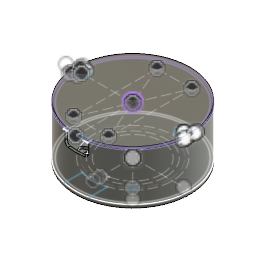
Pixelmapping_gehaeuse (Autodesk Fusion 360 design; units mm, degrees)
Autodesk Fusion 360 part; units mm, degrees
sketch "LED-Ring" plane through (0, 0, 0) normal (0, 1, 0) x (1, 0, 0)
  circle A0 centre (0, 0) radius 18
  circle A1 centre (0, 0) radius 20.7 construction
  line L0 (0, 0) -> (0, -20.7) construction
  line L1 (2.8, -17.9) -> (-2.8, -17.9)
  line L2 (-2.8, -17.9) -> (-2.8, -23.5)
  line L3 (-2.8, -23.5) -> (2.8, -23.5)
  line L4 (2.8, -23.5) -> (2.8, -17.9)
  line L5 (2.8, -17.9) -> (-2.8, -23.5) construction
  line L6 (-2.8, -17.9) -> (2.8, -23.5) construction
  circle A2 centre (0, -20.7) radius 1.75
  line L7 (0, 0) -> (22.6032, -22.6032) construction
  line L8 (0, 0) -> (31.9658, 0) construction
  circle A3 centre (0, 0) radius 23.18 construction
  circle A4 centre (16.3907, -16.3907) radius 1.25
  circle A5 centre (0, 0) radius 36
  circle A6 centre (16.3907, -16.3907) radius 2.25
  line L9 (7.9114, -23.7152) -> (7.9114, -35.1199)
  line L10 (-7.9114, -35.1199) -> (-7.9114, -23.7152)
  arc A7 (-7.9114, -23.7152) -> (7.9114, -23.7152) centre (0, 0) ccw
  arc A8 (17.6777, -17.6777) -> (16.6799, -18.6221) centre (0, 0) ccw
  line L11 (-2.8, -23.5) -> (2.8, -23.5)
  line L12 (2.8, -23.5) -> (2.8, -25.3)
  line L13 (2.8, -25.3) -> (-2.8, -25.3)
  line L14 (-2.8, -25.3) -> (-2.8, -23.5)
  circle A9 centre (0, 0) radius 34.5
  point P0 (0, -20.7)
  point P1 (0, -25)
  dimension "d170" = 50
  dimension "d171" = 36
  dimension "d172" = 2.7
  dimension "d173" = 5.6
  dimension "d174" = 5.6
  dimension "d175" = 3.5
  dimension "d176" = 45
  dimension "d178" = 2.5
  dimension "d179" = 72
  dimension "d190" = 4.5
  dimension "d267" = 1.8
  dimension "d308" = 69
  constraint coincident A0.centre A1.centre
  constraint concentric A0 A8
  constraint coincident A1 P0
  constraint vertical L0
  constraint horizontal L1
  constraint perpendicular L1 L2
  constraint parallel L1 L3
  constraint parallel L2 L4
  constraint coincident L5 P0
  constraint coincident L6 P0
  constraint coincident P0 L0.end
  constraint horizontal L8
  constraint coincident L7 A4.centre
  constraint coincident A3 A4.centre
  constraint concentric A5 A8
  constraint concentric A4 A6
  constraint parallel L9 L10
  constraint coincident P1 A8
  constraint coincident L9.start A8
  constraint coincident L10.end A8
  constraint coincident A5 L10.start
  constraint coincident A5 L9.end
  constraint coincident A6 A8.end
  constraint concentric A3 A8
  constraint coincident L7 A8.start
  constraint horizontal L11
  constraint vertical L12
  constraint horizontal L13
  constraint vertical L14
  constraint concentric A5 A9
  measures "d170" diameter of A8
  measures "d171" diameter of A0
  measures "d173" distance of L2.end L3.end
  measures "d174" distance of L1.end L2.end
  measures "d175" diameter of A2
  measures "d176" angle of L7 L8
  measures "d178" diameter of A4
  measures "d179" diameter of A5
  measures "d190" diameter of A6
  measures "d267" distance of L2.end L13.end
  measures "d308" diameter of A9
extrude "LED-Ring Base Plate" add sketch "LED-Ring" against normal blind 2 contours A0 L1 | A0 L1 L2 L4 A6 A7 A8 L12 L14 | A0 L1 | A0 L1 L2 L3 L4 L11 | L3 A7 A8 L11 L12 L14 | L9 L10 A7 A8 L12 L13 L14 A9 | A7 A8 L12 L13 L14 | A6 L9 L10 A8 A9 | A5 L9 L10 A9 | A5 L9 L10 A9 | A6 | A2 | A4 makes body 1
extrude "Lichtloch" cut sketch "LED-Ring" against normal blind 2 contours A2 bodies 1
pattern_circular "Löcher Lattern" count 12 over 360 about axis through (0, 0, 0) along (0, 1, 0) of "Lichtloch"
extrude "SMD Loch" cut sketch "LED-Ring" against normal blind 1.5 contours A0 L1 | A0 L1 L2 L3 L4 L11 | L3 A7 A8 L11 L12 L14 | A7 A8 L12 L13 L14 picked at (-0.2109, -17.9296) bodies 1
fillet "Fillet4" radius 1.6 2 edges at (2.8, -0.75, 25.3) (-2.8, -0.75, 25.3) on bodies 1
pattern_circular "SMD Aussparungen" count 12 over 360 about axis through (0, 0, 0) along (0, 1, 0) of "SMD Loch", "Fillet4"
extrude "Schraubenloch" cut sketch "LED-Ring" against normal blind 5 contours A4 bodies 1
chamfer "Chamfer4" distance 1 angle 45 1 edges at (15.2253, -2, 16.8428) on bodies 1
pattern_circular "C-Pattern3" count 4 over 360 about axis through (0, 0, 0) along (0, 1, 0) of "Schraubenloch", "Chamfer4"
extrude "Extrude21" cut sketch "LED-Ring" against normal blind 1.4 contours L9 L10 A7 A8 L12 L13 L14 A9 | A7 A8 L12 L13 L14 | A5 L9 L10 A9 picked at (2.2129, -34.8904) bodies 1
extrude "Extrude35" add sketch "LED-Ring" along normal blind 30 and the other way blind 2 contours A5 L9 L10 A9 | A5 L9 L10 A9 bodies 1
sketch "Sketch14" plane through (0, 30, 0) normal (0, 1, 0) x (-1, 0, 0)
  circle A0 centre (0, 0) radius 34.5
  circle A1 centre (0, 0) radius 36
  line L0 (11, 26.25) -> (-11, 26.25) construction
  line L1 (-11, 26.25) -> (-11, -26.25) construction
  line L2 (-11, -26.25) -> (11, -26.25) construction
  line L3 (11, -26.25) -> (11, 26.25) construction
  line L4 (11, 26.25) -> (-11, -26.25) construction
  line L5 (-11, 26.25) -> (11, -26.25) construction
  circle A2 centre (-11, 26.25) radius 1.4
  circle A3 centre (11, 26.25) radius 1.4
  circle A4 centre (-11, -26.25) radius 1.4
  circle A5 centre (11, -26.25) radius 1.4
  line L6 (0, 0) -> (0, 36) construction
  line L7 (0, 0) -> (42, 0) construction
  circle A6 centre (32.2153, 0) radius 1.7
  line L8 (30.5895, 2.7946) -> (28.9822, -0.0107)
  line L9 (28.9822, -0.0107) -> (30.608, -2.8053)
  line L10 (30.608, -2.8053) -> (33.8412, -2.7946)
  line L11 (33.8412, -2.7946) -> (35.4485, 0.0107)
  line L12 (35.4485, 0.0107) -> (33.8226, 2.8053)
  line L13 (33.8226, 2.8053) -> (30.5895, 2.7946)
  line L14 (33.8226, 2.8053) -> (32.2061, 2.8)
  line L15 (35.8908, 2.8019) -> (33.8226, 2.8053)
  line L16 (33.8412, -2.7946) -> (32.2246, -2.8)
  line L17 (35.8919, -2.7879) -> (33.8412, -2.7946)
  line L18 (35.8933, 4.3019) -> (33.8214, 4.3053)
  line L19 (33.8214, 4.3053) -> (29.7185, 4.2918)
  line L20 (29.7185, 4.2918) -> (27.2501, -0.0164)
  line L21 (27.2501, -0.0164) -> (29.747, -4.3082)
  line L22 (29.747, -4.3082) -> (33.8461, -4.2946)
  line L23 (35.8969, -4.2878) -> (33.8461, -4.2946)
  circle A7 centre (32.2153, 0) radius 3.25 construction
  line L24 (-35.8933, -4.3019) -> (-33.8214, -4.3053)
  line L25 (-33.8214, -4.3053) -> (-29.7185, -4.2918)
  line L26 (-29.7185, -4.2918) -> (-27.2501, 0.0164)
  line L27 (-27.2501, 0.0164) -> (-29.747, 4.3082)
  line L28 (-29.747, 4.3082) -> (-33.8461, 4.2946)
  line L29 (-35.8969, 4.2878) -> (-33.8461, 4.2946)
  line L30 (-33.8226, -2.8053) -> (-30.5895, -2.7946)
  line L31 (-30.5895, -2.7946) -> (-28.9822, 0.0107)
  line L32 (-30.608, 2.8053) -> (-33.8412, 2.7946)
  line L33 (-28.9822, 0.0107) -> (-30.608, 2.8053)
  circle A8 centre (-32.2153, 0) radius 1.7
  circle A9 centre (-32.2153, 0) radius 3.25 construction
  line L34 (-35.4485, -0.0107) -> (-33.8226, -2.8053)
  line L35 (-33.8412, 2.7946) -> (-35.4485, -0.0107)
  line L36 (-35.8919, 2.7879) -> (-33.8412, 2.7946)
  line L37 (-35.8908, -2.8019) -> (-33.8226, -2.8053)
  circle A10 centre (0, 0) radius 34.5
  circle A11 centre (0, 0) radius 36
  line L38 (0, 36) -> (-7.5, 36)
  line L39 (-7.5, 36) -> (-7.5, 33.5838)
  line L40 (-7.5, 33.5838) -> (0, 33.5838)
  line L41 (0, 33.5838) -> (0, 36)
  line L42 (0, 36) -> (7.5, 36)
  line L43 (7.5, 36) -> (7.5, 33.6275)
  line L44 (7.5, 33.6275) -> (0, 33.6275)
  line L45 (0, 33.6275) -> (0, 36)
  circle A12 centre (-11, 26.25) radius 2
  circle A13 centre (11, 26.25) radius 2
  circle A14 centre (-11, -26.25) radius 2
  circle A15 centre (11, -26.25) radius 2
  point P0 (32.2153, 0)
  dimension "d313" = 22
  dimension "d314" = 52.5
  dimension "d315" = 2.8
  dimension "d316" = 2.8
  dimension "d317" = 2.8
  dimension "d318" = 2.8
  dimension "d319" = 3.4
  dimension "d320" = 2.8
  dimension "d321" = -1.5
  dimension "d322" = 6.5
  dimension "d334" = 360
  dimension "d341" = 7.5
  dimension "d342" = 7.5
  dimension "d347" = 0.6
  dimension "d348" = 0.6
  dimension "d349" = 0.6
  dimension "d350" = 0.6
  constraint horizontal L0
  constraint perpendicular L0 L1
  constraint parallel L0 L2
  constraint parallel L1 L3
  constraint coincident L4 A0.centre
  constraint coincident L5 A0.centre
  constraint coincident A0.centre A1.centre
  constraint coincident L0.end L1.start
  constraint coincident L0.start L3.end
  constraint coincident L1.end L2.start
  constraint coincident L2.end L3.start
  constraint coincident A1 L6.end
  constraint vertical L6
  constraint horizontal L7
  constraint coincident L7 P0
  constraint coincident P0 A6.centre
  constraint parallel L13 L14
  constraint parallel L10 L16
  constraint parallel L10 L17
  constraint coincident A1 L15.start
  constraint coincident A1 L17.start
  constraint horizontal L38
  constraint vertical L39
  constraint horizontal L40
  constraint vertical L41
  constraint horizontal L42
  constraint vertical L43
  constraint horizontal L44
  constraint vertical L45
  measures "d313" distance of L1.end L2.end
  measures "d314" distance of L0.end L1.end
  measures "d315" diameter of A2
  measures "d316" diameter of A3
  measures "d317" diameter of A4
  measures "d318" diameter of A5
  measures "d319" diameter of A6
  measures "d320" distance of P0 L13
  measures "d322" diameter of A7
  measures "d341" distance of L6.end L38.end
  measures "d342" distance of L6.end L42.end
extrude "Extrude36" add sketch "Sketch14" against normal blind 6.5 contours A0 L8 L9 L10 L11 L12 L13 L14 L16 A10 | A0 L12 L15 A10 | A0 L11 L17 A10 | A0 L8 L9 L10 L13 L14 L15 L16 L17 L18 L19 L20 L21 L22 L23 A10 | A0 L24 L25 L26 L27 L28 L29 L30 L31 L32 L33 L36 L37 A10 | A0 L34 L37 A10 | A0 L30 L31 L32 L33 L34 L35 A10 | A0 L35 L36 A10 | A6 | A8 bodies 1
extrude "Extrude37" cut sketch "Sketch14" against normal blind 2.5 from surface at -2 contours A0 L8 L9 L10 L11 L12 L13 L14 L16 A10 | A0 L11 L12 A10 | A0 L12 L15 A10 | A0 A1 L11 L12 L15 L17 A10 A11 | A0 L11 L17 A10 | A0 A1 L34 L35 L36 L37 A10 A11 | A0 L34 L37 A10 | A0 L34 L35 A10 | A0 L30 L31 L32 L33 L34 L35 A10 | A0 L35 L36 A10 bodies 1
chamfer "Chamfer7" distance 7.23 angle 45 2 edges at (-34.5, 23.5, 0.0057) (34.5, 23.5, -0.0057) on bodies 1
extrude "Extrude38" cut sketch "Sketch14" against normal blind 14 contours A6 | A8 bodies 1
extrude "Extrude39" add sketch "Sketch14" along normal blind 1.5 separate body contours A0 L8 L9 L10 L11 L12 L13 L14 L16 A10 | A0 L11 L12 A10 | A0 L12 L15 A10 | A0 A1 L11 L12 L15 L17 A10 A11 | A0 L11 L17 A10 | A0 L8 L9 L10 L13 L14 L15 L16 L17 L18 L19 L20 L21 L22 L23 A10 | A0 A1 L15 L18 A10 A11 | A0 A1 L17 L23 A10 A11 | A0 L18 L19 L20 L21 L22 L23 L24 L25 L26 L27 L28 L29 A10 L39 L40 L41 L43 L44 | A0 A1 L18 A10 A11 L43 | A0 A1 L23 L24 A10 A11 | A0 A10 L41 L43 L44 L45 | A0 A1 A10 A11 L41 L43 L45 | A0 A1 L24 L37 A10 A11 | A0 L24 L25 L26 L27 L28 L29 L30 L31 L32 L33 L36 L37 A10 | A0 A10 L39 L40 L41 L45 | A0 A1 A10 A11 L39 L41 L45 | A0 A1 L34 L35 L36 L37 A10 A11 | A0 L34 L37 A10 | A0 A1 L29 A10 A11 L39 | A0 L34 L35 A10 | A0 L30 L31 L32 L33 L34 L35 A10 | A0 A1 L29 L36 A10 A11 | A0 L35 L36 A10 | A12 | A13 | A14 | A15 makes body 2
extrude "Extrude41" add sketch "Sketch14" against normal blind 5.6 contours A12 | A13 | A14 | A15 bodies 2
fillet "Fillet6" radius 3 4 edges at (12.8647, 30, 25.5268) (-9.1353, 30, 25.5268) (12.8647, 30, -26.9732) (-9.1353, 30, -26.9732) on bodies 2
chamfer "Chamfer8" distance 1.5 angle 45 2 edges at (-30.6304, 31.5, 0.6147) (33.8003, 31.5, 0.6147) on bodies 2
chamfer "Chamfer9" distance 1.3 angle 45 4 edges at (12.3053, 31.5, 26.7563) (-9.6947, 31.5, 26.7563) (-9.6947, 31.5, -25.7437) (12.3053, 31.5, -25.7437) on bodies 2
extrude "Extrude40" cut sketch "Sketch14" against normal blind 9 contours A0 A1 A10 A11 L41 L43 L45 | A0 A1 A10 A11 L39 L41 L45 bodies 1
fillet "Fillet5" radius 2.5 2 edges at (-7.5, 21, 34.4425) (7.5, 21, 34.4425) on bodies 1
named bodies: "LED-Ring"
